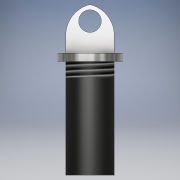
# Autodesk Inventor part: Part1
Saved by Autodesk Inventor 2019 (Build 230136000, 136)
## iProperties
Created: 2021-05-13
Part Number: Part1
Material: Steel, Alloy
Document SubType Name: Modeling
Designer: HP
Density: 7.73 g/cm^3
Appearance: Semi-Polished
Mass: 462.63 g
Surface Area: 128.313 cm^2
Volume: 59.8486 cm^3
Author: HP
Autodesk Inventor part; units mm, degrees
ref_plane "YZ Plane" through (0, 0, 0) normal (1, 0, 0) x (0, 1, 0)
ref_plane "XZ Plane" through (0, 0, 0) normal (0, 1, 0) x (-1, 0, 0)
ref_plane "XY Plane" through (0, 0, 0) normal (0, 0, 1) x (1, 0, 0)
sketch "Sketch1" plane through (0, 0, 0) normal (0, 0, 1) x (1, 0, 0)
  line L0 (0, 0) -> (0, 75)
  line L1 (0, 75) -> (20, 75)
  line L2 (20, 75) -> (20, 70)
  line L3 (20, 70) -> (15, 70)
  line L4 (15, 70) -> (15, 0)
  line L5 (0, 0) -> (15, 0)
  dimension "d0" = 75
  dimension "d1" = 20
  dimension "d2" = 5
  dimension "d3" = 5
  constraints: 12 end point, 3 vertical, 2 perpendicular, 1 horizontal
  measures "d0" distance of L0.start L0.end
  measures "d1" distance of L0.end L1.end
  measures "d2" distance of L1.end L2.end
  measures "d3" distance of L2.end L3.end
revolve "Revolution1" add sketch "Sketch1" angle 360 about axis through (0, 0, 0) along (0, 1, 0)
sketch "Sketch2" plane through (0, 0, 0) normal (0, -1, 0) x (1, 0, 0)
  circle A0 centre (0, 0) radius 12.5
  dimension "d5" = 25
  constraints: 1 centre point, 1 coincident
  measures "d5" diameter of A0
extrude "Extrusion1" cut sketch "Sketch2" against normal blind 50
sketch "Sketch3" plane through (0, 0, 0) normal (0, -1, 0) x (1, 0, 0)
  circle A0 centre (0, 0) radius 12.5
  circle A1 centre (0, 0) radius 7.5
  dimension "d8" = 25
  dimension "d9" = 15
  constraints: 2 centre point, 2 coincident
  measures "d8" diameter of A0
  measures "d9" diameter of A1
extrude "Extrusion2" add sketch "Sketch3" against normal blind 50
sketch "Sketch4" plane through (0, 0, 0) normal (0, 0, 1) x (1, 0, 0)
  line L0 (-20, 75) -> (20, 75) projected
  line L1 (14.924, 75) -> (14.924, 85)
  arc A0 (14.924, 85) -> (1.6102, 104.5279) centre (-4.7241, 85.9067) ccw
  line L2 (-14.924, 75) -> (-14.924, 85)
  arc A1 (-1.6102, 104.5279) -> (-14.924, 85) centre (4.7241, 85.9067) ccw
  arc A2 (1.6102, 104.5279) -> (-1.6102, 104.5279) centre (0, 99.7942) ccw
  circle A3 centre (0, 94.794) radius 7
  line L3 (-14.924, 75) -> (14.924, 75)
  point P0 (0, 0)
  dimension "d14" = 10
  dimension "d15" = 19.669
  dimension "d17" = 5
  dimension "d18" = 14
  constraints: 6 end point, 6 point on circle, 4 centre point, 2 tangent, 1 collinear, 1 perpendicular, 1 point on line
  measures "d14" distance of L1.start L1.end
  measures "d15" radius of A0
  measures "d17" radius of A2
  measures "d18" diameter of A3
extrude "Extrusion3" add sketch "Sketch4" along normal mid plane 10
thread "Thread1" size "M30x3.5" class "6g" standard "ANSI Metric M Profile" length 10 offset 60
body "Solid1"
